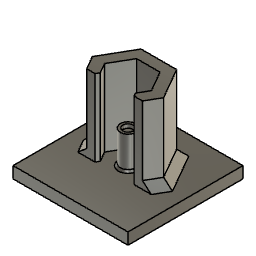
Pin-holder-for-assembly v8 (Autodesk Fusion 360 design; units mm, degrees)
Autodesk Fusion 360 part; units mm, degrees
sketch "Sketch1" plane through (0, 0, 0) normal (0, 0, 1) x (1, 0, 0)
  line L0 (15, 15) -> (-15, 15)
  line L1 (-15, 15) -> (-15, -15)
  line L2 (-15, -15) -> (15, -15)
  line L3 (15, -15) -> (15, 15)
  line L4 (15, 15) -> (-15, -15) construction
  line L5 (-15, 15) -> (15, -15) construction
  dimension "d1" = 30
  dimension "d2" = 30
  constraint horizontal L0
  constraint perpendicular L0 L1
  constraint parallel L0 L2
  constraint parallel L1 L3
  constraint coincident L4 origin
  constraint coincident L5 origin
  measures "d1" distance of L0 L2
  measures "d2" distance of L1 L3
extrude "Extrude1" add sketch "Sketch1" along normal blind 3
sketch "Sketch2" plane through (0, 0, 3) normal (0, 0, 1) x (-1, 0, 0)
  line L0 (-15, 15) -> (-15, -15)
  line L1 (-15, -15) -> (15, -15)
  line L2 (15, -15) -> (15, 15)
  line L3 (15, 15) -> (-15, 15)
  circle A0 centre (0, 0) radius 2
  dimension "d5" = 4
  constraint coincident A0.centre origin
  measures "d5" diameter of A0
extrude "Extrude2" add sketch "Sketch2" along normal blind 8.5 contours A0
sketch "Sketch3" plane through (0, 0, 11.5) normal (0, 0, 1) x (-1, 0, 0)
  circle A0 centre (0, 0) radius 2
  circle A1 centre (0, 0) radius 1.35
  dimension "d8" = 2.7
  constraint concentric A0 A1
  measures "d8" diameter of A1
extrude "Extrude3" cut sketch "Sketch3" against normal blind 1 contours A1
sketch "Sketch4" plane through (0, 0, 3) normal (0, 0, 1) x (-1, 0, 0)
  circle A0 centre (0, 0) radius 2
  line L0 (-15, 15) -> (-15, -15)
  line L1 (-15, -15) -> (15, -15)
  line L2 (15, -15) -> (15, 15)
  line L3 (15, 15) -> (-15, 15)
  line L4 (3.06, -5.3) -> (6.1199, 0)
  line L5 (6.1199, 0) -> (3.06, 5.3)
  line L6 (3.06, 5.3) -> (-3.06, 5.3)
  line L7 (-3.06, 5.3) -> (-6.1199, 0)
  line L8 (-6.1199, 0) -> (-3.06, -5.3)
  line L9 (-3.06, -5.3) -> (3.06, -5.3)
  line L10 (9.2953, 0) -> (4.6477, 8.05)
  line L11 (4.6477, 8.05) -> (-4.6477, 8.05)
  line L12 (-4.6477, 8.05) -> (-9.2953, 0)
  line L13 (-9.2953, 0) -> (-4.6477, -8.05)
  line L14 (-4.6477, -8.05) -> (4.6477, -8.05)
  line L15 (4.6477, -8.05) -> (9.2953, 0)
  line L16 (15, 3.5) -> (-15, 3.5)
  dimension "d11" = 10.5
  dimension "d12" = 2.75
  dimension "d13" = 3.5
  constraint coincident A0.centre origin
  constraint horizontal L9
  constraint coincident L2 L16.start
  constraint coincident L0 L16.end
  constraint perpendicular L0 L16
  measures "d13" distance of L7.end L16
extrude "Extrude4" add sketch "Sketch4" along normal blind 20 contours L4 L5 L7 L8 L9 L10 L12 L13 L14 L15 L16
chamfer "Chamfer1" distance 1 angle 45 2 edges at (4.0992, -3.5, 13) (-4.0992, -3.5, 13)
chamfer "Chamfer2" distance 2 angle 45 3 edges at (6.9715, 4.025, 3) (0, 8.05, 3) (-6.9715, 4.025, 3)
chamfer "Chamfer2" distance 2 angle 45 2 edges at (8.285, -1.75, 3) (-8.285, -1.75, 3)
chamfer "Chamfer2" distance 0.5 angle 45 1 edges at (1.8647, -0.7232, 3)
